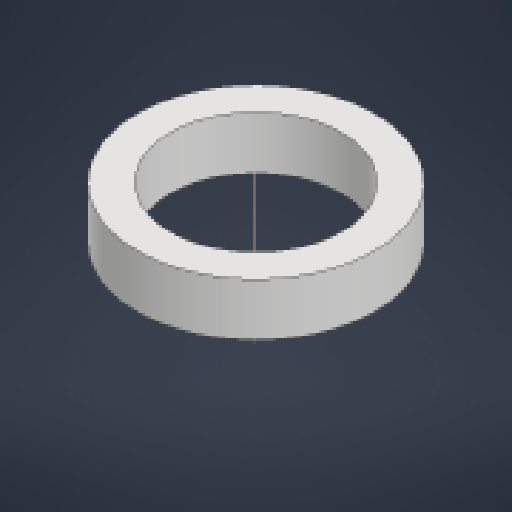
# Autodesk Inventor part: counter_bearing_guide_ring
Saved by Autodesk Inventor 2024 (Build 280153000, 153)
## iProperties
Created: 2026-03-30
Part Number: counter_bearing_guide_ring
Material: Generic
Document SubType Name: Modeling
Designer: schar
Density: 1 g/cm^3
Appearance: Default
Author: schar
Autodesk Inventor part; units mm, degrees
ref_plane "YZ Plane" through (0, 0, 0) normal (1, 0, 0) x (0, 1, 0)
ref_plane "XZ Plane" through (0, 0, 0) normal (0, 1, 0) x (-1, 0, 0)
ref_plane "XY Plane" through (0, 0, 0) normal (0, 0, 1) x (1, 0, 0)
sketch "Sketch1" plane through (0, 0, 0) normal (0, 0, 1) x (1, 0, 0)
  line L0 (-3.3092, 2.2934) -> (-3.3092, 6.2934)
  line L1 (-3.3092, 6.2934) -> (-16.3092, 6.2934) projected
  line L2 (-9.8092, 6.2934) -> (-0.8092, 6.2934)
  line L3 (-0.8092, 6.2934) -> (-3.3092, 6.2934)
  line L4 (-3.3092, 6.2934) -> (-3.3092, 2.2934)
  line L5 (-3.3092, 2.2934) -> (-0.8092, 2.2934)
  line L6 (-0.8092, 2.2934) -> (-0.8092, 6.2934)
  line L7 (-9.8092, 6.2934) -> (-9.8092, 1.9036)
  point P0 (0, 0)
  dimension "d0" = 9
  constraints: 14 end point, 2 horizontal, 2 parallel, 2 vertical, 1 coincident, 1 midpoint, 1 perpendicular, 2 other
  measures "d0" distance of L2.start L2.end
revolve "Revolution1" add sketch "Sketch1" angle 360 about axis through (-9.8092, 6.2934, 0) along (0, -1, 0)
body "Solid1"
